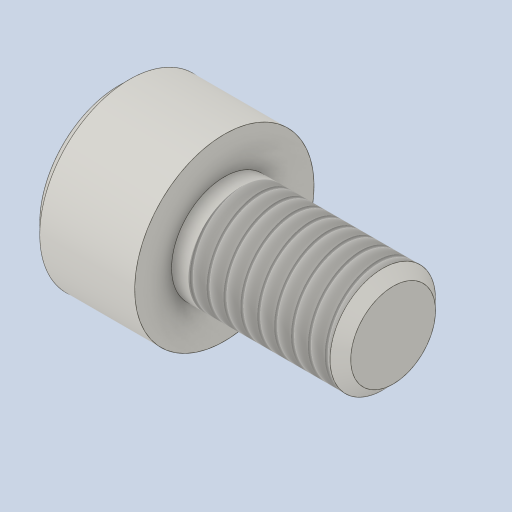
# Autodesk Inventor part: SCB5-8
Saved by Autodesk Inventor 2023 (Build 270158000, 158)
## iProperties
Category: PARTsolutions
Company: MISUMI
Created: 2024-11-11
Part Number: SCB5-8
Material: 鋼
Catalog Web Link: www.cadenas.de
Description: SCB-Hexagon Socket Head Cap Screws - Stainless Steel
Vendor: MISUMI
Document SubType Name: Modeling
Designer: psAdmin
Manufacturer: MISUMI
Mass: 3.13173 g
Surface Area: 3.94783 cm^2
Volume: 0.398946 cm^3
Density: 7.85 g/cm^3
Appearance: 鋼
PSOL_IDENT_0: {$CADENAS_DATA/23d-libs/misumi/metric/27_screws_nuts/scb_fa.prj},151 {VTYP=3D},{NB=SCB5-8},{LINA=SCB
PSOL_IDENT_1: 5-8},{NN=SCB},{DATE=03.06.2021 03:35:43},{GEOMDATE=23.02.2012 00:00:00},{VERSION=},{LINEID=40},{WBVA
PSOL_IDENT_2: R=L},{WBNUMERIC=L}  {NB=SCB5-8},{LINA=SCB5-8},{KT=DUMMY},{PN=SCB5-8},{MAT=SUSXM7(30430 Stainless Ste
PSOL_IDENT_3: el)},{SC=A2-70},{M=5},{L=8},{LL=Full Thread},{L1=22},{TYPE=SCB},{M1=5.0},{L0=6,8,10,12,14,15,16,18,2
PSOL_IDENT_4: 0,22,25,30,35,40,45,50},{MP=5x0.8},{P=0.8},{A=8.5},{E=5.0},{B=4.0},{V=0.50}
NB: SCB5-8
NN: SCB
NT: Hexagon Socket Head Cap Screws - Stainless Steel
NBSYN: $PN.
LINA: SCB5-8
CATALOG: Misumi
PN: SCB5-8
MAT: 302HQ Stainless Steel
SC: A2-70
M: 5
L: 8
LL: Full Thread
MP: 5x0.8
A: 8.5
E: 5
B: 4
SUPPLIER: MISUMI
ARTICLENO: SCB5-8
BOMINFO: SCB5-8
CREATOR: CADENAS GmbH
Title: SCB5-8
Author: Cadenas PARTsolutions
Comments: Hexagon Socket Head Cap Screws - Stainless Steel
Autodesk Inventor part; units mm, degrees
sketch "Sketch_1" plane through (0, 0, 0) normal (0, 0, 1) x (1, 0, 0)
  line L0 (8, 0) -> (-5, 0)
  line L1 (-5, 0) -> (-5, 3.75)
  line L2 (-5, 3.75) -> (-4.5, 4.25)
  line L3 (-4.5, 4.25) -> (0, 4.25)
  line L4 (0, 4.25) -> (0, 2.5)
  line L5 (0, 2.5) -> (7.5095, 2.5)
  line L6 (7.5095, 2.5) -> (8, 2.0095)
  line L7 (8, 2.0095) -> (8, 0)
  line L8 (8, 0) -> (-5, 0)
  constraints: 18 end point
revolve "Revolution1" add sketch "Sketch_1" angle 360 about axis through (8, 0, 0) along (1, 0, 0)
thread "Thread1" size "M5x0.8" class "6g" standard "ISO Metric profile" length 6.7095
sketch "Sketch2" plane through (-5, 0, 0) normal (-1, 0, 0) x (0, 0, 1)
  point P0 (0, 0)
hole "Hole1" at (-5, 0, 0) direction (1, 0, 0) diameter 4 depth 2.5 tip angle 150
sketch "Sketch_3" plane through (-5, 0, 0) normal (1, 0, 0) x (0, 0, -1)
  line L0 (-2, -1.1547) -> (0, -2.3094)
  line L1 (0, -2.3094) -> (2, -1.1547)
  line L2 (2, -1.1547) -> (2, 1.1547)
  line L3 (2, 1.1547) -> (0, 2.3094)
  line L4 (0, 2.3094) -> (-2, 1.1547)
  line L5 (-2, 1.1547) -> (-2, -1.1547)
  constraints: 12 end point
extrude "Extrusion1" cut sketch "Sketch_3" along normal blind 2.5
ref_plane "bolt_XY" through (0, 0, 0) normal (1, 0, 0) x (0, 0, -1)
ref_plane "bolt_YZ" through (0, 0, 0) normal (0, 0, -1) x (0, 1, 0)
ref_plane "bolt_ZX" through (0, 0, 0) normal (0, 1, 0) x (1, 0, 0)
ref_plane "nut_XY" through (8, 0, 0) normal (1, 0, 0) x (0, 0, -1)
ref_plane "nut_YZ" through (8, 0, 0) normal (0, 0, -1) x (0, 1, 0)
ref_plane "nut_ZX" through (8, 0, 0) normal (0, 1, 0) x (1, 0, 0)
body "Solid1"
